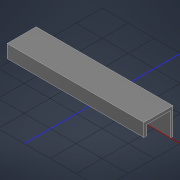
# Autodesk Inventor part: Door_Handle
Saved by Autodesk Inventor 2022.2 (Build 262287010, 287A)
## iProperties
Created: 2022-02-05
Part Number: Door_Handle
Material: ABS-Kunststoff
Document SubType Name: Modeling
Designer: sleib
Density: 1.06 g/cm^3
Appearance: Glatt - Schwarz
Author: sleib
Autodesk Inventor part; units mm, degrees
ref_plane "YZ Plane" through (0, 0, 0) normal (1, 0, 0) x (0, 1, 0)
ref_plane "XZ Plane" through (0, 0, 0) normal (0, 1, 0) x (-1, 0, 0)
ref_plane "XY Plane" through (0, 0, 0) normal (0, 0, 1) x (1, 0, 0)
sketch "Skizze1" plane through (0, 0, 0) normal (0, 0, 1) x (1, 0, 0)
  line L0 (-52.5, -10.25) -> (52.5, -10.25)
  line L1 (52.5, -10.25) -> (52.5, 10.25)
  line L2 (52.5, 10.25) -> (-52.5, 10.25)
  line L3 (-52.5, 10.25) -> (-52.5, -10.25)
  line L4 (-52.5, -10.25) -> (52.5, 10.25) construction
  line L5 (52.5, -10.25) -> (-52.5, 10.25) construction
  line L6 (-52.5, 0) -> (52.5, 0) construction
  circle A0 centre (-22.5, 0) radius 2.75
  circle A1 centre (22.5, 0) radius 2.75
  line L7 (0, -14.35) -> (0, 14.35) construction
  point P0 (0, 0)
  dimension "d0" = 105
  dimension "d1" = 20.5
  dimension "d2" = 5.5
  dimension "d3" = 5.5
  dimension "d4" = 45
  constraints: 14 end point, 4 midpoint, 2 centre point, 2 parallel, 2 point on line, 1 horizontal, 1 perpendicular, 1 symmetric about line
  measures "d0" distance of L2.end L1.end
  measures "d1" distance of L1.end L0.end
  measures "d2" diameter of A0
  measures "d3" diameter of A1
  measures "d4" distance of A1.centre A0.centre
sketch "Skizze2" plane through (0, 0, 0) normal (1, 0, 0) x (0, 1, 0)
  line L0 (-14.35, 0) -> (14.35, 0) construction
  line L1 (0.25, 0) -> (10.25, 0)
  line L2 (10.25, 0) -> (10.25, 20.5)
  line L3 (10.25, 20.5) -> (0.25, 20.5)
  line L4 (0.25, 20.5) -> (0.25, 0)
  line L5 (0.25, 0) -> (7.85, 0)
  line L6 (7.85, 0) -> (7.85, 18.1)
  line L7 (7.85, 18.1) -> (0.25, 18.1)
  line L8 (0.25, 18.1) -> (0.25, 0)
  point P0 (0, 0)
  point P1 (10.25, 0)
  point P2 (0.25, 18.1)
  dimension "d5" = 20.5
  dimension "d6" = 2.4
  dimension "d7" = 2.4
  dimension "d12" = 10
  constraints: 16 end point, 4 parallel, 2 horizontal, 2 perpendicular
  measures "d5" distance of L3.end L1.start
  measures "d6" distance between parallel lines of L6 L2
  measures "d7" distance between parallel lines of L7 L3
  measures "d12" distance between parallel lines of L4 L2
extrude "Extrusion1" add sketch "Skizze1" against normal blind 1.8
extrude "Extrusion2" add sketch "Skizze2" along normal mid plane 105 contours L6 L7 L4 L3 L2 L1
equation "\"d7\" = d6"
equation "\"d10\" = d0"
